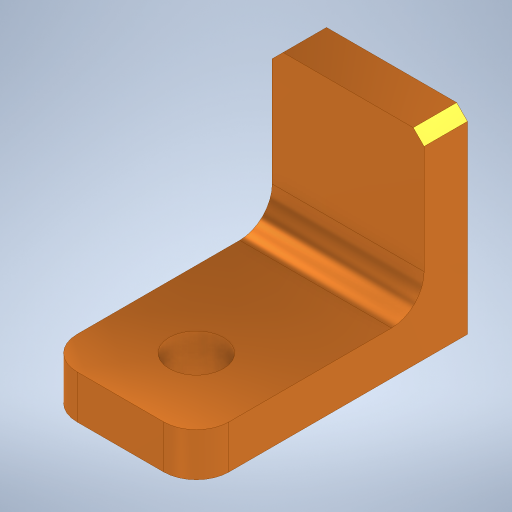
# Autodesk Inventor part: Packa
Saved by Autodesk Inventor 2024.2 (Build 282272000, 272)
## iProperties
Created: 2025-06-02
Part Number: Packa
Material: Zlatá
Document SubType Name: Modeling
Designer: Elite
Density: 19.3 g/cm^3
Appearance: Kov – teplota 1600 F
Mass: 40.7818 g
Surface Area: 15.0069 cm^2
Volume: 2.11305 cm^3
Author: Elite
Autodesk Inventor part; units mm, degrees
ref_plane "YZ Plane" through (0, 0, 0) normal (1, 0, 0) x (0, 1, 0)
ref_plane "XZ Plane" through (0, 0, 0) normal (0, 1, 0) x (-1, 0, 0)
ref_plane "XY Plane" through (0, 0, 0) normal (0, 0, 1) x (1, 0, 0)
sketch "Náčrt1" plane through (0, 0, 0) normal (0, 0, 1) x (1, 0, 0)
  line L0 (0, 0) -> (14, 0)
  line L1 (14, 0) -> (14, 25)
  line L2 (14, 25) -> (0, 25)
  line L3 (0, 25) -> (0, 0)
  circle A0 centre (7, 7) radius 2.5
  point P0 (7, 0)
  dimension "d0" = 14
  dimension "d1" = 25
  dimension "d2" = 5
  dimension "d3" = 7
  dimension "d4" = 7
  constraints: 8 end point, 2 parallel, 1 centre point, 1 horizontal, 1 midpoint, 1 perpendicular
  measures "d0" distance of L2.end L1.end
  measures "d1" distance of L1.end L0.end
  measures "d2" diameter of A0
  measures "d3" distance from line of L3 A0.centre
  measures "d4" distance of point (7, 0) A0.centre
extrude "Vysunutí1" add sketch "Náčrt1" against normal blind 4
sketch "Náčrt2" plane through (0, 0, 0) normal (0, 0, 1) x (1, 0, 0)
  line L0 (0, 0) -> (0, 25) projected
  line L1 (14, 25) -> (14, 0) projected
  line L2 (0, 25) -> (14, 25)
  line L3 (14, 25) -> (14, 21)
  line L4 (14, 21) -> (0, 21)
  line L5 (0, 21) -> (0, 25)
  point P0 (0, 21)
  dimension "d7" = 4
  constraints: 8 end point, 2 parallel, 1 horizontal, 1 perpendicular, 1 point on line
  measures "d7" distance of L2.end L3.end
extrude "Vysunutí2" add sketch "Náčrt2" along normal blind 14
fillet "Zaoblení1" radius 3 1 edges at (7, 21, 0)
fillet "Zaoblení2" radius 3 2 edges at (0, 0, -2) (14, 0, -2)
chamfer "Zkosení1" distance 1 angle 45 2 edges at (0, 23, 14) (14, 23, 14)
